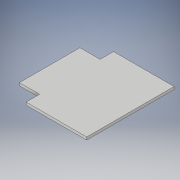
# Autodesk Inventor part: Plate 2
Saved by Autodesk Inventor 2019.4 (Build 234330000, 330)
## iProperties
Created: 2019-11-29
Part Number: Plate 2
Material: Generic
Document SubType Name: Modeling
Designer: admin
Density: 1 g/cm^3
Appearance: Default
Author: admin
Autodesk Inventor part; units mm, degrees
ref_plane "YZ Plane" through (0, 0, 0) normal (1, 0, 0) x (0, 1, 0)
ref_plane "XZ Plane" through (0, 0, 0) normal (0, 1, 0) x (-1, 0, 0)
ref_plane "XY Plane" through (0, 0, 0) normal (0, 0, 1) x (1, 0, 0)
sketch "Sketch1" plane through (0, 0, 0) normal (0, 1, 0) x (-1, 0, 0)
  line L0 (-45, 65) -> (45, 65)
  line L1 (45, 65) -> (45, -65)
  line L2 (45, -65) -> (-45, -65)
  line L3 (-45, -65) -> (-45, 65)
  line L4 (-45, 65) -> (45, -65) construction
  line L5 (45, 65) -> (-45, -65) construction
  line L6 (-45, 45) -> (75, 45)
  line L7 (75, 45) -> (75, -45)
  line L8 (75, -45) -> (-45, -45)
  line L9 (-45, -45) -> (-45, 45)
  line L10 (0, 0) -> (75, 0) construction
  dimension "d0" = 90
  dimension "d1" = 130
  dimension "d2" = 90
  dimension "d3" = 120
  constraints: 22 end point, 4 parallel, 3 horizontal, 3 midpoint, 2 perpendicular, 1 point on line
  measures "d0" distance of L1.end L2.end
  measures "d1" distance of L0.end L1.end
  measures "d2" distance of L6.end L7.end
  measures "d3" distance of L7.end L8.end
extrude "Extrusion1" add sketch "Sketch1" along normal blind 4
body "Solid1"
